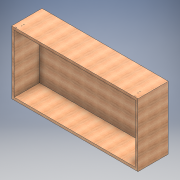
# Autodesk Inventor part: Base
Saved by Autodesk Inventor 2017 (Build 210142000, 142)
## iProperties
Created: 2016-11-26
Part Number: Base
Material: Wood (Birch)
Document SubType Name: Modeling
Designer: umr
Density: 0.55 g/cm^3
Appearance: Birch - Natural Polished
Author: umr
Autodesk Inventor part; units mm, degrees
ref_plane "YZ Plane" through (0, 0, 0) normal (1, 0, 0) x (0, 1, 0)
ref_plane "XZ Plane" through (0, 0, 0) normal (0, 1, 0) x (-1, 0, 0)
ref_plane "XY Plane" through (0, 0, 0) normal (0, 0, 1) x (1, 0, 0)
sketch "Sketch1" plane through (0, 0, 0) normal (0, 1, 0) x (-1, 0, 0)
  line L0 (0, 0) -> (2500, 0)
  line L1 (2500, 0) -> (2500, -1250)
  line L2 (2500, -1250) -> (0, -1250)
  line L3 (0, -1250) -> (0, 0)
  dimension "d0" = 2500
  dimension "d1" = 1250
  constraints: 8 end point, 2 parallel, 1 horizontal, 1 perpendicular
  measures "d0" distance of L1.end L2.end
  measures "d1" distance of L0.end L1.end
extrude "Extrusion1" add sketch "Sketch1" along normal blind 600
sketch "Sketch2" plane through (0, 0, 0) normal (0, -1, 0) x (1, 0, 0)
  line L0 (-50, -50) -> (-2450, -50)
  line L1 (-2450, -50) -> (-2450, -1200)
  line L2 (-2450, -1200) -> (-50, -1200)
  line L3 (-50, -1200) -> (-50, -50)
  line L4 (0, 0) -> (-2500, 0) projected
  line L5 (0, -1250) -> (0, 0) projected
  dimension "d4" = 2400
  dimension "d5" = 1150
  dimension "d8" = 50
  dimension "d9" = 50
  dimension "d10" = 2500
  dimension "d11" = 1250
  constraints: 8 end point, 2 parallel, 1 horizontal, 1 perpendicular
  measures "d4" distance of L2.end L1.end
  measures "d5" distance of L1.end L0.end
  measures "d8" distance between parallel lines of L0 L4
  measures "d9" distance between parallel lines of L5 L3
  measures "d10" distance of L4.start L4.end
  measures "d11" distance of L5.start L4.start
extrude "Extrusion2" cut sketch "Sketch2" against normal blind 500
sketch "Sketch3" plane through (-2500, 0, 0) normal (0, 0, 1) x (1, 0, 0)
  line L0 (2500, 0) -> (0, 0) projected
  line L1 (2500, 0) -> (2500, 600) projected
  line L2 (0, 0) -> (0, 600) projected
  circle A0 centre (2440, 18) radius 3
  circle A1 centre (2420, 18) radius 3
  circle A2 centre (2400, 100) radius 4.25
  circle A3 centre (2400, 140.5) radius 4.25
  dimension "d12" = 6
  dimension "d13" = 18
  dimension "d14" = 60
  dimension "d20" = 6
  dimension "d21" = 18
  dimension "d23" = 20
  dimension "d24" = 8.5
  dimension "d25" = 8.5
  dimension "d26" = 100
  dimension "d27" = 40.5
  dimension "d28" = 100
  dimension "d29" = 100
  constraints: 4 centre point
  measures "d12" diameter of A0
  measures "d13" distance from line of L0 A0.centre
  measures "d14" distance from line of L1 A0.centre
  measures "d20" diameter of A1
  measures "d21" distance from line of L0 A1.centre
  measures "d23" distance of A1.centre A0.centre
  measures "d24" diameter of A2
  measures "d25" diameter of A3
  measures "d26" distance from line of A2.centre L0
  measures "d27" distance of A3.centre A2.centre
  measures "d28" distance from line of L1 A2.centre
  measures "d29" distance from line of L1 A3.centre
extrude "Extrusion3" cut sketch "Sketch3" against normal blind 10
ref_plane "Work Plane1" through (-2500, 0, -625) normal (0, 0, 1) x (1, 0, 0)
mirror "Mirror1" about plane through (-2500, 0, -625) normal (0, 0, 1) of "Extrusion3"
ref_plane "Work Plane2" through (-1250, 0, -1250) normal (-1, 0, 0) x (0, 0, 1)
mirror "Mirror2" about plane through (-1250, 0, -1250) normal (-1, 0, 0) of "Extrusion3"
mirror "Mirror3" about plane through (-2500, 0, -625) normal (0, 0, 1) of "Mirror2", "Extrusion3"
equation "\"d4\" = d10 - 2 * d9"
equation "\"d5\" = d11 - 2 * d8"
equation "\"d9\" = d8"
equation "\"d13\" = 3 * d12"
equation "\"d21\" = d13"
equation "\"d29\" = d28"
body "Solid1"
